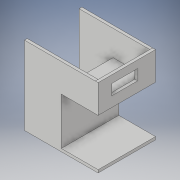
# Autodesk Inventor part: sanicav
Saved by Autodesk Inventor 2018 (Build 220112000, 112)
## iProperties
Created: 2021-04-16
Part Number: sanicav
Material: Generic
Document SubType Name: Modeling
Designer: Joel Olguin Lopez
Density: 1 g/cm^3
Appearance: Default
Author: Joel Olguin Lopez
Autodesk Inventor part; units mm, degrees
ref_plane "YZ Plane" through (0, 0, 0) normal (1, 0, 0) x (0, 1, 0)
ref_plane "XZ Plane" through (0, 0, 0) normal (0, 1, 0) x (-1, 0, 0)
ref_plane "XY Plane" through (0, 0, 0) normal (0, 0, 1) x (1, 0, 0)
sketch "Boceto1" plane through (0, 0, 0) normal (0, 1, 0) x (-1, 0, 0)
  line L0 (-16.5612, -12.9032) -> (16.5612, -12.9032)
  line L1 (16.5612, -12.9032) -> (16.5612, 12.9032)
  line L2 (16.5612, 12.9032) -> (-16.5612, 12.9032)
  line L3 (-16.5612, 12.9032) -> (-16.5612, -12.9032)
  line L4 (-16.5612, -12.9032) -> (16.5612, 12.9032) construction
  line L5 (16.5612, -12.9032) -> (-16.5612, 12.9032) construction
  point P0 (0, 0)
  dimension "d0" = 16.5612
  dimension "d1" = 12.9032
  constraints: 12 end point, 2 midpoint, 2 parallel, 1 horizontal, 1 perpendicular
  measures "d0" distance from line of L1 point (0, 0)
  measures "d1" distance from line of point (0, 0) L0
extrude "Extrusión1" add sketch "Boceto1" along normal blind 1.27
sketch "Boceto2" plane through (-16.5612, 0, 12.9032) normal (0, 0, 1) x (1, 0, 0)
  line L0 (0, 1.27) -> (0, 35.1613)
  line L1 (0, 35.1613) -> (33.1216, 35.1613)
  line L2 (33.1216, 35.1613) -> (33.1216, 22.4613)
  line L3 (33.1216, 22.4613) -> (16.5608, 22.4613)
  line L4 (16.5608, 22.4613) -> (16.5612, 1.27)
  line L5 (33.1224, 1.27) -> (0, 1.27) projected
  point P0 (16.5612, 0)
  dimension "d4" = 33.1216
  dimension "d5" = 12.7
  dimension "d6" = 16.5608
  dimension "d7" = 21.1913
  constraints: 10 end point, 2 perpendicular, 1 horizontal, 1 midpoint, 1 vertical
  measures "d4" distance of L0.end L1.end
  measures "d5" distance of L1.end L2.end
  measures "d6" distance of L2.end L3.end
  measures "d7" distance of L3.end L4.end
extrude "Extrusión2" add sketch "Boceto2" against normal blind 1.27
mirror "Simetría1" about plane through (0, 0, 0) normal (0, 0, 1) of "Extrusión2"
sketch "Boceto3" plane through (-0.0004, 22.4613, -11.6332) normal (1, 0, 0) x (0, 0, -1)
  line L0 (0, -21.191) -> (-23.2664, -21.191) projected
  line L1 (-23.2664, -21.191) -> (-23.2664, -0.0276)
  line L2 (-23.2664, -0.0276) -> (0, -0.0276)
  line L3 (0, 0) -> (0, -21.1913) projected
  line L4 (0, -0.0276) -> (0, -21.1913)
  line L5 (0, -21.1913) -> (-23.2664, -21.191)
  point P0 (-11.6332, -22.4613)
  dimension "d10" = 21.1634
  constraints: 8 end point, 1 collinear, 1 perpendicular, 1 vertical
  measures "d10" distance of L0.end L1.end
extrude "Extrusión3" add sketch "Boceto3" against normal blind 1.27
sketch "Boceto4" plane through (-0.0004, 22.4337, 11.6332) normal (0, 1, 0) x (1, 0, 0)
  line L0 (16.561, 23.2664) -> (16.5608, 23.2664) projected
  line L1 (16.561, -1.27) -> (-1.2701, -1.27)
  line L2 (-1.27, 0) -> (-1.27, 23.2664) projected
  line L3 (-1.2701, -1.27) -> (-1.2701, 24.5364)
  line L4 (16.5612, 24.5364) -> (-16.5612, 24.5364) projected
  line L5 (-1.2701, 24.5364) -> (16.5612, 24.5364)
  line L6 (16.5612, 24.5364) -> (16.561, -1.27)
  dimension "d23" = 17.8312
  constraints: 8 end point, 1 collinear, 1 parallel, 1 perpendicular
  measures "d23" distance of L1.start L1.end
extrude "Extrusión4" add sketch "Boceto4" along normal blind 1.27
sketch "Boceto7" plane through (16.5606, 22.434, 12.9032) normal (1, 0, 0) x (0, 0, -1)
  line L0 (0, 0) -> (25.8062, 0)
  line L1 (25.8062, -22.4334) -> (25.8062, 12.7279) projected
  line L2 (25.8062, 12.7279) -> (0, 12.7279)
  line L3 (0, 12.7279) -> (0, 0)
  line L4 (0, 1.27) -> (25.8064, 1.27) projected
  dimension "d28" = 1.27
  dimension "d29" = 25.8062
  constraints: 6 end point, 2 horizontal, 1 perpendicular, 1 point on line
  measures "d28" distance between parallel lines of L4 L0
  measures "d29" distance of L0.start L0.end
extrude "Extrusión7" add sketch "Boceto7" against normal blind 1.27
sketch "Boceto8" plane through (16.5606, 22.434, 12.9032) normal (1, 0, 0) x (0, 0, -1)
  line L0 (6.1467, 9.3592) -> (17.78, 9.3592)
  line L1 (17.78, 9.3592) -> (17.78, 4.572)
  line L2 (17.78, 4.572) -> (6.1467, 4.572)
  line L3 (6.1467, 4.572) -> (6.1467, 9.3592)
  line L4 (25.8064, 0) -> (0, 0) projected
  line L5 (0, 12.7273) -> (0, 1.27) projected
  point P0 (12.9031, -22.4337)
  dimension "d30" = 4.7871
  dimension "d31" = 11.6333
  dimension "d36" = 4.572
  dimension "d37" = 17.78
  constraints: 8 end point, 2 parallel, 1 horizontal, 1 perpendicular
  measures "d30" distance of L0.end L1.end
  measures "d31" distance of L0.start L0.end
  measures "d36" distance between parallel lines of L4 L2
  measures "d37" distance between parallel lines of L5 L1
extrude "Extrusión8" cut sketch "Boceto8" against normal up to next
sketch "Boceto9" plane through (-0.0004, 22.4337, 11.6332) normal (0, -1, 0) x (1, 0, 0)
  circle A0 centre (8.2804, -3.5112) radius 2.3532
  line L0 (0, -24.5364) -> (0, 1.27) projected
  line L1 (15.291, 0) -> (-1.2701, 0) projected
  point P0 (0, -11.6332)
  dimension "d42" = 4.7064
  dimension "d43" = 8.2804
  dimension "d44" = 3.5112
  constraints: 1 centre point
  measures "d42" diameter of A0
  measures "d43" distance from line of L0 A0.centre
  measures "d44" distance from line of L1 A0.centre
extrude "Extrusión9" cut sketch "Boceto9" against normal up to next
sketch "Boceto10" plane through (0, 1.27, 12.9032) normal (1, 0, 0) x (0, 0, -1)
  circle A0 centre (23.114, 10.5788) radius 1.0858
  circle A1 centre (20.574, 10.5788) radius 1.0858
  line L0 (0, -0.0003) -> (25.8064, -0.0003) projected
  line L1 (0, 21.1637) -> (0, 0) projected
  point P0 (12.9032, -1.27)
  dimension "d47" = 2.1716
  dimension "d48" = 10.5791
  dimension "d49" = 23.114
  dimension "d50" = 2.54
  dimension "d51" = 10.5791
  constraints: 2 centre point, 1 equal radius
  measures "d47" diameter of A0
  measures "d48" distance from line of L0 A0.centre
  measures "d49" distance from line of L1 A0.centre
  measures "d50" distance of A1.centre A0.centre
  measures "d51" distance from line of A1.centre L0
extrude "Extrusión10" cut sketch "Boceto10" against normal up to next
